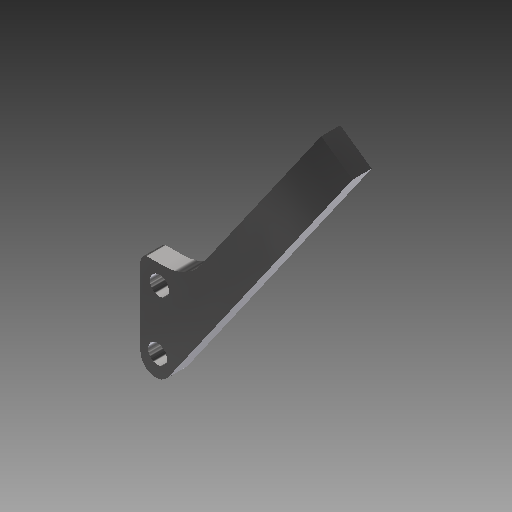
# Autodesk Inventor part: Dźwignia
Saved by Autodesk Inventor 2017 (Build 210142000, 142)
## iProperties
Created: 2015-12-05
Part Number: Dźwignia
Material: Stal nierdzewna
Document SubType Name: Sheet Metal
Designer: graaapsik
Density: 8.08 g/cm^3
Sheet Metal Rule: Default_mm
Appearance: Częściowo polerowany
Mass: 37.9547 g
Surface Area: 30.2612 cm^2
Volume: 4.69736 cm^3
Author: graaapsik
Autodesk Inventor part; units mm, degrees
ref_plane "YZ Plane" through (0, 0, 0) normal (1, 0, 0) x (0, 1, 0)
ref_plane "XZ Plane" through (0, 0, 0) normal (0, 1, 0) x (-1, 0, 0)
ref_plane "XY Plane" through (0, 0, 0) normal (0, 0, 1) x (1, 0, 0)
sketch "Szkic1" plane through (0, 0, 0) normal (0, 0, 1) x (1, 0, 0)
  line L0 (0, 0) -> (0, 35)
  line L1 (0, 35) -> (12.2995, 35)
  line L2 (25, 35.7037) -> (0, 0)
  line L3 (25, 35.7037) -> (55.5014, 79.2642)
  line L4 (51.404, 82.1333) -> (51.404, 82.1333)
  line L5 (47.3099, 85) -> (12.2995, 35)
  arc A0 (25, 35.7037) -> (25, 35.7037) centre (22.5425, 37.4244) ccw
  line L6 (47.3099, 85) -> (55.5014, 79.2642)
  point P0 (0, 0)
  point P1 (0, 17.4345)
  dimension "d0" = 10
  dimension "d1" = 35
  dimension "d3" = 50
  dimension "d7" = 25
  dimension "d10" = 35
  measures "d0" distance between parallel lines of L5 L3
  measures "d1" distance of L0.end point (0, 0)
  measures "d3" distance from line of L5.start L1
  measures "d7" distance from line of L3.start L0
  measures "d10" angle of L0 L5
extrude "Płyta1" add sketch "Szkic1" along normal blind 5 contours A0 | L0 L1 L5 L6 L3 L2
sketch "Szkic2" plane through (0, 0, 0) normal (0, 0, 1) x (1, 0, 0)
  line L0 (0, 35) -> (12.2995, 35) construction
  line L1 (0, 0) -> (0, 35) construction
  line L2 (55.5014, 79.2642) -> (0, 0) construction
  point P0 (4.5, 14.2722)
  point P1 (5, 30)
  dimension "d12" = 5
  dimension "d13" = 5
  dimension "d14" = 4.5
  dimension "d15" = 4.5
  measures "d12" distance from line of L0 point (5, 30)
  measures "d13" distance from line of L1 point (5, 30)
  measures "d14" distance from line of L1 point (4.5, 14.272)
  measures "d15" distance from line of L2 point (4.5, 14.272)
hole "Otwór1" at (4.5, 14.2722, 0) at (5, 30, 0) direction (0, 0, 1) diameter 5 end through all
fillet "Zaokrąglenie2" radius 2 1 edges at (0, 35, 2.5)
fillet "Zaokrąglenie3" radius 12 1 edges at (12.2995, 35, 2.5)
fillet "Zaokrąglenie4" radius 4 1 edges at (0, 0, 2.5)
equation "\"d21\" = Grubość"
equation "\"PromieńGięcia\" = Grubość"
equation "\"SzerokośćGięciaPodcięcia\" = Grubość"
equation "\"GłębokośćGięciaPodcięcia\" = 0.5 * Grubość"
equation "\"PromieńPrzejścia\" = PromieńGięcia"
equation "\"Rozmiar_promienia_Jacobiego\" = PromieńGięcia"
equation "\"Wielk_odstępu\" = Grubość"
equation "\"d11\" = PromieńGięcia"
equation "\"Grubość\" = 5"
